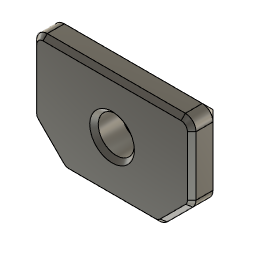
[a]_Railstops_x6 (Autodesk Fusion 360 design; units mm, degrees)
Autodesk Fusion 360 part; units mm, degrees
sketch "Sketch1" plane through (0, 0, 0) normal (0, 1, 0) x (1, 0, 0) in component "[a]_Railstops_x6"
  line L0 (7.5, 5) -> (-7.5, 5)
  line L1 (-7.5, 5) -> (-7.5, -5)
  line L2 (-7.5, -5) -> (7.5, -5)
  line L3 (7.5, -5) -> (7.5, 5)
  line L4 (7.5, 5) -> (-7.5, -5) construction
  line L5 (-7.5, 5) -> (7.5, -5) construction
  dimension "d1" = 15
  dimension "d2" = 10
  constraint horizontal L0
  constraint perpendicular L0 L1
  constraint parallel L0 L2
  constraint parallel L1 L3
  constraint coincident L4 origin
  constraint coincident L5 origin
  measures "d1" distance of L1.end L2.end
  measures "d2" distance of L0.end L1.end
extrude "Extrude1" add sketch "Sketch1" along normal mid plane 3 in component "[a]_Railstops_x6"
chamfer "Chamfer1" distance 3 angle 45 2 edges at (-7.5, 0, -5) (7.5, 0, -5) measured on face at (-2.5, 0.5, -5) measured on face at (7.5, -0.5, 1.6667) in component "[a]_Railstops_x6"
fillet "Fillet1" radius 1 6 edges at (7.5, 0, 5) (-7.5, 0, 5) (-7.5, 0, -2) (-4.5, 0, -5) (4.5, 0, -5) (7.5, 0, -2) in component "[a]_Railstops_x6"
chamfer "Chamfer2" distance 0.4 angle 45 1 faces at (-1.3619, -1.5, 1.6667) in component "[a]_Railstops_x6"
chamfer "Chamfer2" distance 1 angle 45 1 faces at (-1.3619, 1.5, 1.6667) in component "[a]_Railstops_x6"
sketch "Sketch2" plane through (0, -1.5, 0) normal (0, -1, 0) x (1, 0, 0) in component "[a]_Railstops_x6"
  arc A0 (6.9243, -2.0101) -> (7.1, -1.5858) centre (6.5, -1.5858) ccw
  line L0 (7.1, -1.5858) -> (7.1, 4)
  arc A1 (7.1, 4) -> (6.5, 4.6) centre (6.5, 4) ccw
  line L1 (6.5, 4.6) -> (-6.5, 4.6)
  arc A2 (-6.5, 4.6) -> (-7.1, 4) centre (-6.5, 4) ccw
  line L2 (-7.1, 4) -> (-7.1, -1.5858)
  arc A3 (-7.1, -1.5858) -> (-6.9243, -2.0101) centre (-6.5, -1.5858) ccw
  line L3 (-6.9243, -2.0101) -> (-4.5101, -4.4243)
  arc A4 (-4.5101, -4.4243) -> (-4.0858, -4.6) centre (-4.0858, -4) ccw
  line L4 (-4.0858, -4.6) -> (4.0858, -4.6)
  arc A5 (4.0858, -4.6) -> (4.5101, -4.4243) centre (4.0858, -4) ccw
  line L5 (4.5101, -4.4243) -> (6.9243, -2.0101)
  line L6 (0, 0) -> (0, 7) construction
  point P0 (0, 0.5)
  dimension "d16" = 0.5
  constraint coincident L6.start origin
  constraint vertical L6
  constraint coincident P0 L6
  measures "d16" distance of L6.start P0
hole "Hole1" at (0, -1.5, 0) direction (0, 1, 0) diameter 3.4 end through all in component "[a]_Railstops_x6"
chamfer "Chamfer3" distance 0.4 angle 45 2 edges at (0.6147, -1.5, 1.585) (-0.6147, 1.5, 1.585) measured on face at (-5.2858, -1.5, 0.9308) measured on face at (4.8858, 1.5, 0.9308) in component "[a]_Railstops_x6"
component "[a]_Railstops_x6" placed x (1, 0, 0) y (0, 1, 0) z (0, 0, 1) at (0, 0, 0)
